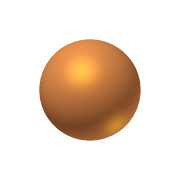
# Autodesk Inventor part: Ball
Saved by Autodesk Inventor 2012 (Build 160160000, 160)
## iProperties
Created: 2012-01-13
Part Number: Ball
Material: Default
Document SubType Name: Modeling
Designer: JesseK
Density: 1 g/cm^3
Author: JesseK
Autodesk Inventor part; units mm, degrees
ref_plane "YZ Plane" through (0, 0, 0) normal (1, 0, 0) x (0, 1, 0)
ref_plane "XZ Plane" through (0, 0, 0) normal (0, 1, 0) x (-1, 0, 0)
ref_plane "XY Plane" through (0, 0, 0) normal (0, 0, 1) x (1, 0, 0)
sketch "Sketch1" plane through (0, 0, 0) normal (0, 0, 1) x (1, 0, 0)
  arc A0 (0, 100.965) -> (0, -100.965) centre (0, 0) ccw
  line L0 (0, 100.965) -> (0, -100.965)
  dimension "d0" = 100.965
  dimension "d0" = 100.965
  constraints: 2 end point, 2 point on circle, 1 centre point, 1 coincident, 1 vertical
  measures "d0" radius of A0
revolve "Revolution1" add sketch "Sketch1" angle 360 about axis through (0, 100.965, 0) along (0, -1, 0)
body "Solid1"
